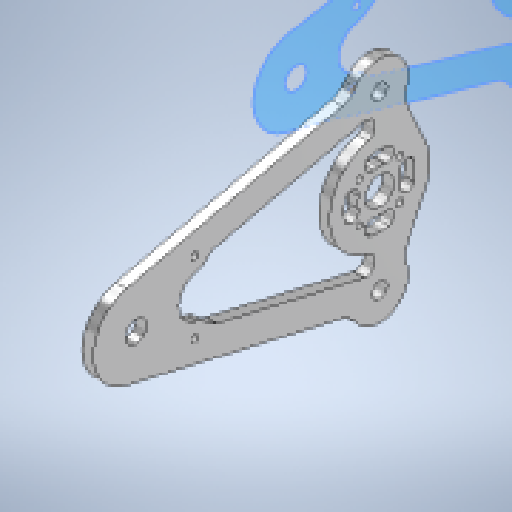
# Autodesk Inventor part: Frame (Motor Side)
Saved by Autodesk Inventor 2023.2 (Build 272271000, 271)
## iProperties
Created: 2022-05-22
Part Number: Frame (Motor Side)
Material: Aluminum 6061
Document SubType Name: Modeling
Designer: Nathan Cai
Density: 2.7 g/cm^3
Appearance: Aluminum - Flat
Mass: 86.2633 g
Surface Area: 157.268 cm^2
Volume: 31.9494 cm^3
Author: Nathan Cai
Autodesk Inventor part; units mm, degrees
ref_plane "YZ Plane" through (0, 0, 0) normal (1, 0, 0) x (0, 1, 0)
ref_plane "XZ Plane" through (0, 0, 0) normal (0, 1, 0) x (-1, 0, 0)
ref_plane "XY Plane" through (0, 0, 0) normal (0, 0, 1) x (1, 0, 0)
sketch "Sketch1" plane through (0, 0, 0) normal (1, 0, 0) x (0, 1, 0)
  circle A0 centre (0, 0) radius 6.35
  circle A1 centre (0, 0) radius 22.225
  line L0 (0, 0) -> (0, 107.95) construction
  circle A2 centre (0, 107.95) radius 4.7625
  circle A3 centre (0, 107.95) radius 76.2 construction
  circle A4 centre (0, 107.95) radius 19.05
  line L1 (0, 0) -> (38.1, 0) construction
  circle A5 centre (38.1, 0) radius 3.3655
  arc A6 (31.9145, -1.4361) -> (35.4542, 5.7725) centre (38.1, 0) ccw
  line L2 (40.7458, -5.7725) -> (9.2604, -20.2038)
  line L3 (18.5565, 112.2582) -> (44.2855, 1.4361)
  line L4 (10.2473, 91.8909) -> (31.9145, -1.4361)
  line L5 (35.4542, 5.7725) -> (22.2231, -0.2919) construction
  circle A7 centre (-38.1, 0) radius 3.3655
  arc A8 (-35.4542, 5.7725) -> (-31.9145, -1.4361) centre (-38.1, 0) ccw
  line L6 (-40.7458, -5.7725) -> (-9.2604, -20.2038)
  line L7 (-18.5565, 112.2582) -> (-44.2855, 1.4361)
  line L8 (-10.2473, 91.8909) -> (-31.9145, -1.4361)
  line L9 (-35.4542, 5.7725) -> (-22.2231, -0.2919)
  line L10 (0, 0) -> (0, -9.5) construction
  line L11 (0, 0) -> (9.5, 0) construction
  line L12 (0, 0) -> (-8, 0) construction
  line L13 (0, 0) -> (-12.5, 0) construction
  line L14 (0, 0) -> (12.7, 0) construction
  line L15 (38.1, 0) -> (15.5821, 96.9909) construction
  circle A9 centre (19.05, 82.0537) radius 1.7526
  circle A10 centre (-19.05, 82.0537) radius 1.7526
  arc A11 (21.6394, 5.0682) -> (29.9543, 7.0072) centre (25.7959, 6.0417) ccw
  arc A12 (-29.9543, 7.0072) -> (-21.6394, 5.0682) centre (-25.7959, 6.0417) ccw
  line L16 (19.05, 82.0537) -> (-19.05, 82.0537) construction
  circle A13 centre (15.875, 82.0537) radius 6.35
  circle A14 centre (15.875, 82.0537) radius 1.7526
  circle A15 centre (-15.875, 82.0537) radius 6.35
  circle A16 centre (-15.875, 82.0537) radius 1.7526
  arc A17 (25.5255, 1.7813) -> (29.4272, 9.2775) centre (38.1, 0) ccw
  arc A18 (-29.4272, 9.2775) -> (-25.5255, 1.7813) centre (-38.1, 0) ccw
  circle A19 centre (0, 0) radius 8 construction
  line L17 (0, 0) -> (5.6569, -5.6569) construction
  circle A20 centre (5.6569, -5.6569) radius 1.5
  circle A21 centre (0, 0) radius 12.5 construction
  circle A22 centre (8.8388, -8.8388) radius 1.5
  circle A23 centre (-6.7175, -6.7175) radius 1.5
  line L18 (-6.7175, -6.7175) -> (0, 0) construction
  circle A24 centre (0, 0) radius 9.5 construction
  circle A25 centre (6.7175, 6.7175) radius 1.5
  circle A26 centre (-5.6569, 5.6569) radius 1.5
  circle A27 centre (-8.8388, 8.8388) radius 1.5
  circle A28 centre (0, 0) radius 16 construction
  circle A29 centre (16, 0) radius 3.5
  circle A30 centre (8, 13.8564) radius 3.5
  circle A31 centre (-8, 13.8564) radius 3.5
  circle A32 centre (-16, 0) radius 3.5
  circle A33 centre (-8, -13.8564) radius 3.5
  circle A34 centre (8, -13.8564) radius 3.5
  point P0 (-9.2604, -20.2038)
  point P1 (30.7423, 3.6129)
  point P2 (-22.2231, -0.2919)
  point P3 (-30.7423, 3.6129)
  point P4 (-10.2473, 91.8909)
  point P5 (-21.6394, 5.0682)
  point P6 (-29.9543, 7.0072)
  point P7 (11.4694, 86.6268)
  point P8 (13.9349, 76.0073)
  point P9 (-13.9349, 76.0073)
  point P10 (-11.4694, 86.6268)
  point P11 (-41.7982, 12.1496)
  point P12 (-30.7475, -10.3552)
  point P13 (30.7475, -10.3552)
  point P14 (41.7982, 12.1496)
  dimension "d58" = 16
  dimension "d61" = 25
  dimension "d65" = 19
  dimension "d70" = 32
  dimension "d0" = 12.7
  dimension "d1" = 44.45
  dimension "d2" = 107.95
  dimension "d3" = 9.525
  dimension "d4" = 152.4
  dimension "d5" = 38.1
  dimension "d6" = 38.1
  dimension "d7" = 6.731
  dimension "d8" = 12.7
  dimension "d9" = 0
  dimension "d10" = 12.7
  dimension "d11" = 12.7
  dimension "d15" = 9.5
  dimension "d16" = 270
  dimension "d18" = 8
  dimension "d20" = 12.5
  dimension "d36" = 3.5052
  dimension "d37" = 19.05
  dimension "d54" = 12.7
  dimension "d55" = 3.5052
  dimension "d56" = 15.875
  dimension "d57" = 25.4
  dimension "d59" = 45
  dimension "d60" = 3
  dimension "d62" = 3
  dimension "d63" = 90
  dimension "d64" = 3
  dimension "d68" = 360
  dimension "d71" = 7
  dimension "d74" = 360
  constraints: 38 end point, 31 centre point, 23 point on circle, 20 symmetric about line, 18 coincident, 7 point on line, 7 tangent, 4 horizontal, 3 parallel, 2 perpendicular, 1 collinear, 1 horizontal alignment, 1 vertical, 44 other
  measures "d0" diameter of A0
  measures "d1" diameter of A1
  measures "d2" distance of L0.start L0.end
  measures "d3" diameter of A2
  measures "d4" diameter of A3
  measures "d5" diameter of A4
  measures "d6" distance of L1.start L1.end
  measures "d7" diameter of A5
  measures "d8" diameter of A6
  measures "d9" distance from line of A0.centre L1
  measures "d10" distance between parallel lines of L3 L4
  measures "d11" distance between parallel lines of L2 L5
  measures "d15" distance of L0.start L10.end
  measures "d18" distance of L0.start L12.end
  measures "d20" distance of L0.start L13.end
  measures "d36" diameter of A9
  measures "d37" distance from line of L0 L16.start
  measures "d54" diameter of A13
  measures "d55" diameter of A14
  measures "d56" distance from line of L0 A14.centre
  measures "d57" diameter of A17
  measures "d59" angle of L11 L17
  measures "d60" diameter of A20
  measures "d62" diameter of A22
  measures "d63" angle of L17 L18
  measures "d64" diameter of A23
  measures "d71" diameter of A29
extrude "Extrusion1" add sketch "Sketch1" along normal blind 4.7625 contours A1 | A1 A11 A17 L2 | A1 L9 A18 A12 | A11 L4 A6 L2 A17 | L6 A18 L9 A1 | L2 A6 L3 A17 | A18 L9 A12 | L4 A17 L3 A6 | A18 L7 A8 L6 | L6 A8 L8 L9 A18 | A17 L4 A13 A4 L3 | L9 L8 A12 | A8 L9 L8 | A18 L8 L9 A8 L7 | L7 A4 L8 A15 A18 | A4 | A13 L4 | L4 A13 | A15 L8 | L8 A15 | A9 A14 | A16 A10 picked at (19.7267, 81.9115) picked at (-19.7267, 82.1959)
fillet "Fillet1" radius 9.525 10 edges at (2.3813, 10.2473, 91.8909) (2.3813, -10.2473, 91.8909) (2.3813, 13.9349, 76.0073) (2.3813, 11.4694, 86.6268) (2.3813, -11.4694, 86.6268) (2.3813, -13.9349, 76.0073) (2.3813, 30.7475, -10.3552) (2.3813, -30.7475, -10.3552) (2.3813, 41.7982, 12.1496) (2.3813, -41.7982, 12.1496)
equation "\"d2\" = C2C"
equation "\"d11\" = d10"
equation "\"d37\" = Leg_Offset"
equation "\"d56\" = Leg_Mounts"
equation "\"C2C\" = 107.95"
equation "\"Leg_Offset\" = 19.05"
equation "\"Leg_Mounts\" = 15.875"
body "Solid1"
